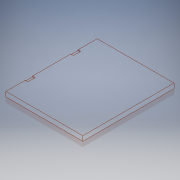
# Autodesk Inventor part: Extension Shelves
Saved by Autodesk Inventor 2016 (Build 200138000, 138)
## iProperties
Created: 2017-10-31
Part Number: Extension Shelves
Material: Wood (Oak)
Document SubType Name: Modeling
Designer: mathaetaes
Density: 0.76 g/cm^3
Appearance: White Oak - Natural Medium Gloss
Author: mathaetaes
Autodesk Inventor part; units mm, degrees
ref_plane "YZ Plane" through (0, 0, 0) normal (1, 0, 0) x (0, 1, 0)
ref_plane "XZ Plane" through (0, 0, 0) normal (0, 1, 0) x (-1, 0, 0)
ref_plane "XY Plane" through (0, 0, 0) normal (0, 0, 1) x (1, 0, 0)
sketch "Sketch1" plane through (0, 0, 0) normal (0, 1, 0) x (-1, 0, 0)
  line L0 (312.1225, 324.0216) -> (-94.2775, 324.0216)
  line L1 (-94.2775, 324.0216) -> (-94.2775, -158.5784)
  line L2 (-94.2775, -158.5784) -> (312.1225, -158.5784)
  line L3 (312.1225, -158.5784) -> (312.1225, 324.0216)
  point P0 (0, 0)
  dimension "d0" = 406.4
  dimension "d1" = 482.6
  constraints: 8 end point, 2 parallel, 1 horizontal, 1 perpendicular
  measures "d0" distance of L1.end L2.end
  measures "d1" distance of L0.end L1.end
extrude "Board" add sketch "Sketch1" along normal blind 25.4
sketch "Hinge Cuts" plane through (0, 25.4, 0) normal (0, 1, 0) x (1, 0, 0)
  line L0 (-312.1225, 158.5784) -> (-312.1225, -324.0216) projected
  line L1 (-312.1225, 56.9784) -> (-300.9973, 56.9784)
  line L2 (-297.8223, 53.8034) -> (-297.8223, 22.0534)
  line L3 (-300.9973, 18.8784) -> (-312.1225, 18.8784)
  line L4 (-312.1225, 18.8784) -> (-312.1225, 56.9784)
  line L5 (94.2775, 158.5784) -> (-312.1225, 158.5784) projected
  line L6 (-312.1225, -222.4216) -> (-300.9973, -222.4216)
  line L7 (-297.8223, -219.2466) -> (-297.8223, -187.4966)
  line L8 (-300.9973, -184.3216) -> (-312.1225, -184.3216)
  line L9 (-312.1225, -184.3216) -> (-312.1225, -222.4216)
  arc A0 (-297.8223, -187.4966) -> (-300.9973, -184.3216) centre (-300.9973, -187.4966) ccw
  arc A1 (-300.9973, -222.4216) -> (-297.8223, -219.2466) centre (-300.9973, -219.2466) ccw
  arc A2 (-300.9973, 18.8784) -> (-297.8223, 22.0534) centre (-300.9973, 22.0534) ccw
  arc A3 (-297.8223, 53.8034) -> (-300.9973, 56.9784) centre (-300.9973, 53.8034) ccw
  point P0 (0, 0)
  point P1 (-297.8223, 18.8784)
  point P2 (-297.8223, 56.9784)
  point P3 (-297.8223, -184.3216)
  point P4 (-297.8223, -222.4216)
  dimension "d4" = 38.1
  dimension "d5" = 14.3002
  dimension "d6" = 101.6
  dimension "d7" = 38.1
  dimension "d8" = 14.3002
  dimension "d9" = 203.2
  dimension "d10" = 3.175
  constraints: 16 end point, 10 point on line, 8 point on circle, 8 tangent, 4 centre point, 4 parallel, 3 equal radius, 2 horizontal, 2 perpendicular
  measures "d4" distance of point (-297.822, 56.978) point (-297.822, 18.878)
  measures "d5" distance of point (-297.822, 18.878) L3.end
  measures "d6" distance between parallel lines of L5 L1
  measures "d7" distance of point (-297.822, -222.422) point (-297.822, -184.322)
  measures "d8" distance of point (-297.822, -184.322) L8.end
  measures "d9" distance between parallel lines of L3 L8
  measures "d10" radius of A0
extrude "Extrusion2" cut sketch "Hinge Cuts" against normal blind 3.175
equation "\"d6\" = 0.25 * d1 - 0.5 * d4"
equation "\"d7\" = d4"
equation "\"d8\" = d5"
equation "\"d9\" = 2 * d6"
body "Solid1"
